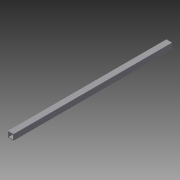
# Autodesk Inventor part: SideLong
Saved by Autodesk Inventor 2013 SP2 (Build 170200200, 200)
## iProperties
Created: 2015-01-07
Part Number: SideLong
Material: Generic
Document SubType Name: Modeling
Designer: darkb_000
Density: 1 g/cm^3
Author: darkb_000
Autodesk Inventor part; units mm, degrees
ref_plane "YZ Plane" through (0, 0, 0) normal (1, 0, 0) x (0, 1, 0)
ref_plane "XZ Plane" through (0, 0, 0) normal (0, 1, 0) x (-1, 0, 0)
ref_plane "XY Plane" through (0, 0, 0) normal (0, 0, 1) x (1, 0, 0)
sketch "Sketch1" plane through (0, 0, 0) normal (0, 0, 1) x (1, 0, 0)
  line L0 (0, 76.2) -> (25.4, 76.2) projected
  line L1 (25.4, 76.2) -> (0, 76.2)
  line L2 (0, 76.2) -> (0, 101.6)
  line L3 (0, 101.6) -> (25.4, 101.6)
  line L4 (25.4, 101.6) -> (25.4, 76.2)
  point P0 (0, 0)
  dimension "d0" = 25.4
  dimension "d1" = 25.4
  constraints: 8 end point, 2 parallel, 1 horizontal, 1 perpendicular
  measures "d0" distance of L2.end L3.end
  measures "d1" distance of L1.end L2.end
ref_plane "Work Plane1" through (0, 0, -711.2) normal (0, 0, -1) x (0, 1, 0)
extrude "Extrusion1" add sketch "Sketch1" against normal up to surface (711.2 mm away)
sketch "Sketch2" plane through (25.4, 76.2, -711.2) normal (0, 0, -1) x (-1, 0, 0)
  line L0 (25.4, 25.4) -> (22.225, 25.4)
  line L1 (22.225, 25.4) -> (22.225, 22.225)
  line L2 (22.225, 22.225) -> (25.4, 22.225)
  line L3 (25.4, 22.225) -> (25.4, 25.4)
  line L4 (0, 0) -> (3.175, 0)
  line L5 (3.175, 0) -> (3.175, 3.175)
  line L6 (3.175, 3.175) -> (0, 3.175)
  line L7 (0, 3.175) -> (0, 0)
  line L8 (3.175, 3.175) -> (22.225, 3.175)
  line L9 (22.225, 3.175) -> (22.225, 22.225)
  line L10 (22.225, 22.225) -> (3.175, 22.225)
  line L11 (3.175, 22.225) -> (3.175, 3.175)
  point P0 (25.4, -76.2)
  dimension "d4" = 3.175
  dimension "d5" = 3.175
  dimension "d6" = 3.175
  dimension "d7" = 3.175
  constraints: 24 end point, 6 parallel, 3 horizontal, 3 perpendicular
  measures "d4" distance of L2.end L1.end
  measures "d5" distance of L1.end L0.end
  measures "d6" distance of L6.end L5.end
  measures "d7" distance of L5.end L4.end
extrude "Extrusion2" cut sketch "Sketch2" against normal through all contours L9 L8 L11 L10
body "Solid1"
